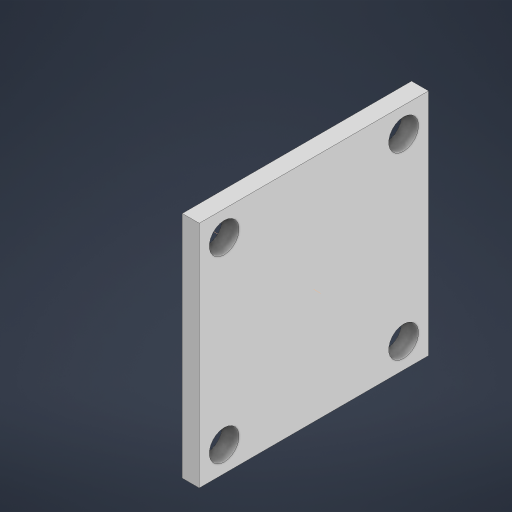
# Autodesk Inventor part: magentic_encoder_modell
Saved by Autodesk Inventor 2024 (Build 280153000, 153)
## iProperties
Created: 2026-03-30
Part Number: magentic_encoder_modell
Material: Generic
Document SubType Name: Modeling
Designer: schar
Density: 1 g/cm^3
Appearance: Default
Author: schar
Autodesk Inventor part; units mm, degrees
ref_plane "YZ Plane" through (0, 0, 0) normal (1, 0, 0) x (0, 1, 0)
ref_plane "XZ Plane" through (0, 0, 0) normal (0, 1, 0) x (-1, 0, 0)
ref_plane "XY Plane" through (0, 0, 0) normal (0, 0, 1) x (1, 0, 0)
sketch "Sketch1" plane through (0, 0, 0) normal (1, 0, 0) x (0, 1, 0)
  line L0 (11.5, 11.5) -> (-11.5, 11.5)
  line L1 (-11.5, 11.5) -> (-11.5, -11.5)
  line L2 (-11.5, -11.5) -> (11.5, -11.5)
  line L3 (11.5, -11.5) -> (11.5, 11.5)
  line L4 (11.5, 11.5) -> (-11.5, -11.5) construction
  line L5 (-11.5, 11.5) -> (11.5, -11.5) construction
  line L6 (11.5, 11.5) -> (11.5, 9)
  line L7 (11.5, 9) -> (9, 9)
  circle A0 centre (9, 9) radius 1.5
  line L8 (11.5, 0) -> (-11.5, 0)
  line L9 (0, 11.5) -> (0, -11.5)
  line L10 (11.5, -11.5) -> (-11.5, 11.5) construction
  line L11 (11.5, -9) -> (9, -9)
  circle A1 centre (9, -9) radius 1.5
  circle A2 centre (-9, 9) radius 1.5
  circle A3 centre (-9, -9) radius 1.5
  point P0 (0, 0)
  dimension "d0" = 23
  dimension "d1" = 23
  dimension "d2" = 2.5
  dimension "d3" = 2.5
  dimension "d4" = 3
  constraints: 24 end point, 6 midpoint, 5 symmetric about line, 4 centre point, 3 point on line, 2 coincident, 2 parallel, 1 horizontal, 1 perpendicular, 3 other
  measures "d0" distance of L2.end L1.end
  measures "d1" distance of L1.end L0.end
  measures "d2" distance of L0.start L6.end
  measures "d3" distance of L6.end L7.end
  measures "d4" diameter of A0
extrude "Extrusion1" add sketch "Sketch1" along normal blind 1.7
ref_plane "Work Plane1" through (0, 0, 11.5) normal (0, 1, 0) x (1, 0, 0)
ref_plane "Work Plane2" through (0, -11.5, 0) normal (0, 0, -1) x (-1, 0, 0)
body "Solid1"
